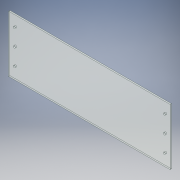
# Autodesk Inventor part: ARM_076_LexanShield
Saved by Autodesk Inventor 2018.3 (Build 223284000, 284)
## iProperties
Created: 2020-02-14
Part Number: ARM_076_LexanShield
Material: Generic
Document SubType Name: Modeling
Designer: 22barlalex
Density: 1 g/cm^3
Appearance: Clear
Author: 22barlalex
Autodesk Inventor part; units mm, degrees
ref_plane "YZ Plane" through (0, 0, 0) normal (1, 0, 0) x (0, 1, 0)
ref_plane "XZ Plane" through (0, 0, 0) normal (0, 1, 0) x (-1, 0, 0)
ref_plane "XY Plane" through (0, 0, 0) normal (0, 0, 1) x (1, 0, 0)
sketch "Sketch1" plane through (0, 0, 0) normal (0, 0, 1) x (1, 0, 0)
  line L0 (0, 0) -> (362.9152, 0)
  line L1 (362.9152, 0) -> (362.9152, 127)
  line L2 (362.9152, 127) -> (0, 127)
  line L3 (0, 127) -> (0, 0)
  dimension "d0" = 362.9152
  dimension "d1" = 127
  constraints: 8 end point, 2 parallel, 1 horizontal, 1 perpendicular
  measures "d0" distance of L2.end L1.end
  measures "d1" distance of L1.end L0.end
extrude "Extrusion1" add sketch "Sketch1" along normal blind 3.175
sketch "Sketch2" plane through (0, 0, 3.175) normal (0, 0, 1) x (1, 0, 0)
  line L0 (0, 127) -> (0, 0) projected
  line L1 (362.9152, 0) -> (362.9152, 127) projected
  line L2 (362.9152, 127) -> (0, 127) projected
  line L3 (0, 0) -> (362.9152, 0) projected
  point P0 (12.7, 25.4)
  point P1 (12.7, 63.5)
  point P2 (350.2152, 25.4)
  point P3 (350.2152, 63.5)
  point P4 (12.7, 101.6)
  point P5 (350.2152, 101.6)
  dimension "d4" = 12.7
  dimension "d5" = 12.7
  dimension "d6" = 12.7
  dimension "d7" = 12.7
  dimension "d8" = 12.7
  dimension "d9" = 12.7
  dimension "d10" = 25.4
  dimension "d11" = 25.4
  dimension "d12" = 38.1
  constraints: 3 horizontal alignment
  measures "d4" distance from line of L0 point (12.7, 25.4)
  measures "d5" distance from line of L0 point (12.7, 63.5)
  measures "d6" distance from line of L1 point (350.215, 25.4)
  measures "d7" distance from line of L1 point (350.215, 63.5)
  measures "d8" distance from line of L0 point (12.7, 101.6)
  measures "d9" distance from line of L1 point (350.215, 101.6)
  measures "d10" distance from line of L2 point (12.7, 101.6)
  measures "d11" distance from line of L3 point (12.7, 25.4)
  measures "d12" distance of point (12.7, 25.4) point (12.7, 63.5)
hole "Hole1" at (12.7, 25.4, 3.175) at (12.7, 63.5, 3.175) at (350.2152, 25.4, 3.175) at (350.2152, 63.5, 3.175) at (12.7, 101.6, 3.175) at (350.2152, 101.6, 3.175) direction (0, 0, -1) diameter 4.8514 end through all
body "Solid1"
